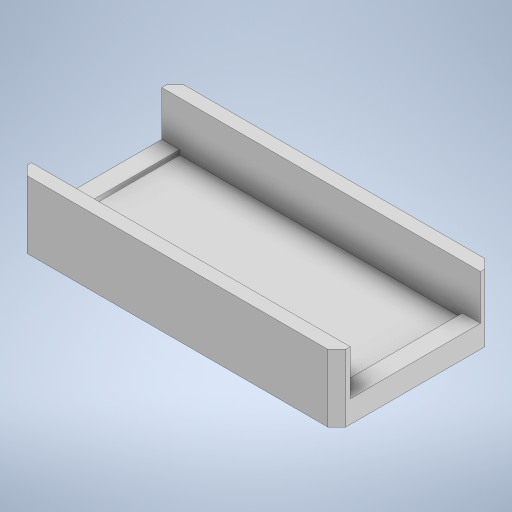
# Autodesk Inventor part: Buck Converter Holder
Saved by Autodesk Inventor 2023 (Build 270158000, 158)
## iProperties
Created: 2026-02-18
Part Number: Buck Converter Holder
Material: Generic
Document SubType Name: Modeling
Designer: Matthew
Density: 1 g/cm^3
Appearance: Default
Author: Matthew
Autodesk Inventor part; units mm, degrees
ref_plane "YZ Plane" through (0, 0, 0) normal (1, 0, 0) x (0, 1, 0)
ref_plane "XZ Plane" through (0, 0, 0) normal (0, 1, 0) x (-1, 0, 0)
ref_plane "XY Plane" through (0, 0, 0) normal (0, 0, 1) x (1, 0, 0)
sketch "Sketch1" plane through (0, 0, 0) normal (0, 1, 0) x (-1, 0, 0)
  line L0 (0, 0) -> (0, -29)
  line L1 (0, 0) -> (65, 0)
  line L2 (65, 0) -> (65, -29)
  line L3 (65, -29) -> (0, -29)
  dimension "d0" = 29
  dimension "d1" = 65
  constraints: 8 end point, 2 perpendicular, 1 horizontal, 1 vertical
  measures "d0" distance of L0.start L0.end
  measures "d1" distance of L0.start L1.end
extrude "Extrusion1" add sketch "Sketch1" along normal blind 4
sketch "Sketch3" plane through (0, 0, 0) normal (0, -1, 0) x (1, 0, 0)
  line L0 (0, 0) -> (0, -29) projected
  line L1 (-65, 0) -> (0, 0) projected
  line L2 (-65, -29) -> (-65, 0) projected
  line L3 (0, -29) -> (-65, -29) projected
  line L4 (3, -32) -> (3, 3)
  line L5 (3, 3) -> (-68, 3)
  line L6 (-68, 3) -> (-68, -32)
  line L7 (-68, -32) -> (3, -32)
  dimension "d4" = 3
  constraints: 8 end point, 3 other
  measures "d4" distance between parallel lines of L0 L4
extrude "Extrusion2" add sketch "Sketch3" against normal blind 15
sketch "Sketch4" plane through (3, 0, 3) normal (1, 0, 0) x (0, 0, -1)
  line L0 (3, 4) -> (32, 4) projected
  line L1 (32, 4) -> (3, 4) projected
  line L2 (3, 4) -> (3, 15)
  line L3 (32, 4) -> (32, 15)
  line L4 (3, 4) -> (32, 4)
  line L5 (3, 15) -> (32, 15)
  line L6 (0, 15) -> (35, 15) projected
  point P0 (3, 0)
  constraints: 8 end point, 2 collinear, 2 vertical
extrude "Extrusion3" cut sketch "Sketch4" against normal blind 72.15
chamfer "Chamfer1" distance 2 angle 45 4 edges at (3, 7.5, 3) (-68, 7.5, 3) (-68, 7.5, -32) (3, 7.5, -32)
sketch "Sketch5" plane through (0, 4, 0) normal (0, 1, 0) x (1, 0, 0)
  line L0 (-68, 0) -> (-68, 29) projected
  line L1 (3, 29) -> (3, 0) projected
  line L2 (-68, 29) -> (3, 29) projected
  line L3 (-1, 29) -> (-1, 0)
  line L4 (-64, 29) -> (-64, 0)
  line L5 (3, 0) -> (-68, 0) projected
  point P0 (0, 0)
  constraints: 4 end point, 3 point on line, 2 vertical
extrude "Extrusion4" add sketch "Sketch5" along normal blind 1 contours L0 L2 L4 L5 | L3 L2 L1 L5
body "Solid1"
